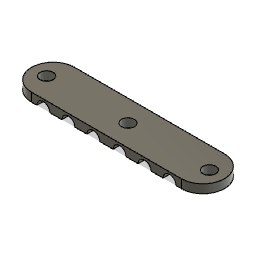
Layout for Electronics board v1 (Autodesk Fusion 360 archive; units mm, degrees)
design "ESc indie mount"
Autodesk Fusion 360 part; units mm, degrees
sketch "Sketch1" plane through (0, 0, 0) normal (0, 0, 1) x (1, 0, 0)
  line L0 (0, 0) -> (17.1, 0)
  line L1 (17.1, 0) -> (17.1, 2)
  line L2 (17.1, 2) -> (0, 2)
  line L3 (0, 2) -> (0, 0)
  line L4 (0, 0) -> (1.25, 0)
  line L5 (1.25, 0) -> (2.75, 0)
  circle A0 centre (2.75, 0) radius 1.5
  line L6 (4.25, 0) -> (7.05, 0)
  line L7 (7.05, 0) -> (8.55, 0)
  circle A1 centre (8.55, 0) radius 1.5
  line L8 (10.05, 0) -> (12.85, 0)
  line L9 (12.85, 0) -> (14.35, 0)
  circle A2 centre (14.35, 0) radius 1.5
  line L10 (15.85, 0) -> (17.1, 0)
  line L11 (15.85, 0) -> (17.4, 0)
  line L12 (17.4, 0) -> (18.95, 0)
  line L13 (18.95, 0) -> (17.1, 0)
  line L14 (17.1, 0) -> (17.1, 2)
  line L15 (17.1, 2) -> (18.95, 2)
  line L16 (18.95, 2) -> (18.95, 0)
  line L17 (17.1, 2) -> (34.2, 2)
  line L18 (34.2, 0) -> (17.1, 0)
  line L19 (18.95, 0) -> (20.45, 0)
  circle A3 centre (20.45, 0) radius 1.5
  line L20 (21.95, 0) -> (24.75, 0)
  line L21 (24.75, 0) -> (26.25, 0)
  circle A4 centre (26.25, 0) radius 1.5
  line L22 (27.75, 0) -> (30.55, 0)
  line L23 (30.55, 0) -> (32.05, 0)
  circle A5 centre (32.05, 0) radius 1.5
  line L24 (33.55, 0) -> (34.8, 0)
  line L25 (34.8, 0) -> (33.05, 0)
  line L26 (33.05, 0) -> (33.05, 2)
  line L27 (33.05, 2) -> (34.8, 2)
  line L28 (34.8, 2) -> (34.8, 0)
  dimension "d1" = 17.1
  dimension "d2" = 2
  dimension "d3" = 1.25
  dimension "d4" = 1.5
  dimension "d5" = 2.8
  dimension "d6" = 1.5
  dimension "d7" = 2.8
  dimension "d8" = 1.5
  dimension "d32" = 1.55
  dimension "d33" = 1.55
  dimension "d39" = 1.5
  dimension "d41" = 2.8
  dimension "d42" = 1.5
  dimension "d43" = 2.8
  dimension "d44" = 1.5
  dimension "d45" = 1.25
  constraint horizontal L0
  constraint vertical L1
  constraint horizontal L2
  constraint vertical L3
  constraint coincident L0.start L3.end
  constraint perpendicular L3 L4
  constraint parallel L0 L5
  constraint coincident L5.end A0.centre
  constraint coincident L4.end A0
  constraint coincident L0 L6.start
  constraint coincident A0 L6.start
  constraint parallel L0 L6
  constraint parallel L0 L7
  constraint coincident L7.end A1.centre
  constraint coincident L6.end A1
  constraint coincident A1 L8.start
  constraint coincident L0 L8.start
  constraint parallel L0 L8
  constraint parallel L0 L9
  constraint coincident L9.end A2.centre
  constraint coincident L8.end A2
  constraint coincident L0 L10.start
  constraint coincident A2 L10.start
  constraint perpendicular L1 L11
  constraint perpendicular L1 L12
  constraint horizontal L13
  constraint vertical L14
  constraint horizontal L15
  constraint vertical L16
  constraint symmetric L0.start L14 L18.start
  constraint symmetric L0.end L14 L1.start
  constraint symmetric L1.end L14 L2.start
  constraint symmetric L2.end L14 L17.end
  constraint perpendicular L16 L19
  constraint coincident L19.end A3.centre
  constraint coincident L12.end A3
  constraint coincident L18 L20.start
  constraint coincident A3 L20.start
  constraint parallel L18 L20
  constraint parallel L18 L21
  constraint coincident L21.end A4.centre
  constraint coincident L20.end A4
  constraint coincident A4 L22.start
  constraint coincident L18 L22.start
  constraint parallel L18 L22
  constraint parallel L18 L23
  constraint coincident L23.end A5.centre
  constraint coincident L22.end A5
  constraint coincident A5 L24.start
  constraint coincident L18 L24.start
  constraint horizontal L25
  constraint vertical L26
  constraint horizontal L27
  constraint vertical L28
  constraint coincident L17 L26.end
  measures "d1" distance of L0.start L0.end
  measures "d2" distance of L0.start L2.end
  measures "d3" distance of L0.start L4.end
  measures "d4" distance of L4.end L5.end
  measures "d5" distance of L6.start L6.end
  measures "d6" distance of L6.end L7.end
  measures "d7" distance of L8.start L8.end
  measures "d8" distance of L8.end L9.end
  measures "d32" distance of L10.start L11.end
  measures "d33" distance of L11.end L12.end
  measures "d39" distance of L12.end L19.end
  measures "d41" distance of L20.start L20.end
  measures "d42" distance of L20.end L21.end
  measures "d43" distance of L22.start L22.end
  measures "d44" distance of L22.end L23.end
  measures "d45" distance of L24.start L24.end
extrude "Extrude1" add sketch "Sketch1" along normal blind 10 contours L0 L1 L2 L3 L4 A0 L6 A1 L8 A2 L10 L11 L14 | L1 L11 L12 L13 L14 L15 L16 L17 L18 | L16 L17 L18 A3 L20 A4 L22 A5 L26 | L17 L18 A5 L24 L25 L26 L27 L28
sketch "Sketch10" plane through (0, 0, 0) normal (0, -1, 0) x (1, 0, 0)
  line L0 (15.85, 0) -> (18.95, 0)
  line L1 (18.95, 0) -> (18.95, 10)
  line L2 (18.95, 10) -> (15.85, 10)
  line L3 (15.85, 10) -> (15.85, 0)
  line L4 (15.85, 0) -> (18.95, 0)
  line L5 (17.4, 0) -> (17.4, 10)
  circle A0 centre (17.4, 5) radius 1.5
  dimension "d46" = 3
  constraint coincident L0.start L3.end
  constraint coincident L0.end L1.start
  constraint midpoint L0 L5.start
  constraint midpoint L2 L5.end
  constraint midpoint L5 A0.centre
  measures "d46" diameter of A0
extrude "Extrude6" cut sketch "Sketch10" against normal blind 2.6 contours L5 A0 | L5 A0
sketch "Sketch7" plane through (0, 2, 0) normal (0, 1, 0) x (-1, 0, 0)
  line L0 (-34.8, 0) -> (0, 0)
  line L1 (0, 0) -> (0, 10)
  line L2 (0, 10) -> (-34.8, 10)
  line L3 (0, 0) -> (0, 10)
  line L4 (0, 0) -> (-34.8, 0)
  line L5 (-17.4, 0) -> (-17.4, 10)
  circle A0 centre (0, 5) radius 5
  line L6 (0, 5) -> (5, 5)
  circle A1 centre (-17.4, 5) radius 1.5
  line L7 (-34.8, 10) -> (-34.8, 0)
  line L8 (2.5, 5) -> (0, 5)
  line L9 (2.5, 5) -> (2.1, 5)
  line L10 (2.5, 5) -> (0.5, 5)
  line L11 (2.5, 5) -> (1, 5)
  line L12 (1, 5) -> (1.5, 5)
  circle A2 centre (1.5, 5) radius 1.5
  circle A3 centre (-34.8, 5) radius 5
  circle A4 centre (-36.3, 5) radius 1.5
  line L13 (0, 10) -> (-1.25, 10)
  line L14 (-1.25, 10) -> (-1.25, 0)
  line L15 (5, 5) -> (-1.25, 5)
  dimension "d49" = 0.4
  dimension "d50" = 2
  dimension "d52" = 0.5
  constraint coincident L0.end L1.start
  constraint coincident L1.end L2.start
  constraint coincident L0.start L4.end
  constraint midpoint L4 L5.start
  constraint midpoint L2 L5.end
  constraint midpoint L3 A0.centre
  constraint coincident L1.end A0
  constraint coincident A0.centre L6.start
  constraint coincident A0 L6.end
  constraint perpendicular L3 L6
  constraint parallel L8 L9
  constraint parallel L8 L10
  constraint coincident L6 L11.end
  constraint parallel L8 L12
  constraint coincident L12.end A2.centre
  constraint coincident A0.centre A2
  constraint symmetric L5 A0 A3
  constraint symmetric L5 A2 A4
  constraint coincident L2 L13.end
  constraint tangent A0 L13
  constraint coincident L4 L14.end
  constraint perpendicular L4 L14
  constraint midpoint L14 L15.end
  constraint perpendicular L14 L15
  measures "d49" distance of L8.start L9.end
  measures "d50" distance of L8.start L10.end
  measures "d52" distance of L11.end L12.end
extrude "Extrude5" add sketch "Sketch7" against normal blind 2 contours L7 A3 | L1 L3 A0 L6 A2 L15 | L1 L3 A0 L6 A2 L15 picked at (-35.3657, 1.2198)
